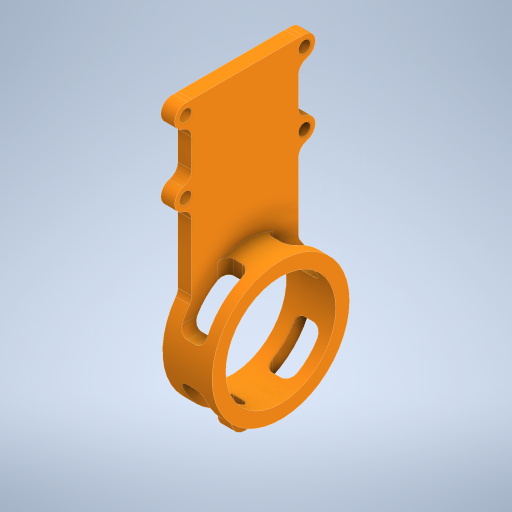
# Autodesk Inventor part: RSFF_cover_2_v2_clearance
Saved by Autodesk Inventor 2023 (Build 270158000, 158)
## iProperties
Created: 2023-10-18
Part Number: RSFF_cover_2_v2_clearance
Material: Generic
Document SubType Name: Modeling
Designer: MichihisaOohara
Density: 1 g/cm^3
Appearance: オレンジ
Author: MichihisaOohara
Autodesk Inventor part; units mm, degrees
ref_plane "YZ Plane" through (0, 0, 0) normal (1, 0, 0) x (0, 1, 0)
ref_plane "XZ Plane" through (0, 0, 0) normal (0, 1, 0) x (-1, 0, 0)
ref_plane "XY Plane" through (0, 0, 0) normal (0, 0, 1) x (1, 0, 0)
sketch "スケッチ1" plane through (0, 0, 0) normal (1, 0, 0) x (0, 1, 0)
  circle A0 centre (0, 0) radius 10
  circle A1 centre (0, 0) radius 12.5
  line L0 (24.5, 10.8) -> (37.5, 10.8)
  line L1 (37.5, 10.8) -> (37.5, -10.8)
  line L2 (37.5, -10.8) -> (24.5, -10.8)
  line L3 (24.5, -10.8) -> (24.5, 10.8)
  circle A2 centre (37.5, 10.8) radius 1.1
  circle A3 centre (37.5, -10.8) radius 1.1
  circle A4 centre (24.5, 10.8) radius 1.1
  circle A5 centre (24.5, -10.8) radius 1.1
  line L4 (0, 9.7) -> (39.5, 9.7)
  line L5 (39.5, 9.7) -> (39.5, -9.7)
  line L6 (39.5, -9.7) -> (0, -9.7)
  line L7 (0, -9.7) -> (0, 9.7)
  circle A6 centre (37.5, 10.8) radius 2
  circle A7 centre (37.5, -10.8) radius 2
  circle A8 centre (24.5, -10.8) radius 2
  circle A9 centre (24.5, 10.8) radius 2
  point P0 (7.8842, 9.7)
  point P1 (7.8842, -9.7)
  point P2 (22.8297, -9.7)
  point P3 (26.1703, -9.7)
  point P4 (35.8297, -9.7)
  point P5 (39.1703, -9.7)
  point P6 (39.1703, 9.7)
  point P7 (35.8297, 9.7)
  point P8 (26.1703, 9.7)
  point P9 (22.8297, 9.7)
  dimension "d0" = 20
  dimension "d1" = 25
  dimension "d2" = 13
  dimension "d3" = 24.5
  dimension "d4" = 10.8
  dimension "d5" = 21.6
  dimension "d6" = 2.2
  dimension "d7" = 2.2
  dimension "d8" = 2.2
  dimension "d9" = 2.2
  dimension "d10" = 19.4
  dimension "d11" = 9.7
  dimension "d12" = 2
  dimension "d13" = 0
  dimension "d14" = 4
  dimension "d15" = 4
  dimension "d16" = 4
  dimension "d17" = 4
  constraints: 16 end point, 10 centre point, 10 coincident, 4 parallel, 2 horizontal, 2 perpendicular
  measures "d0" diameter of A0
  measures "d1" diameter of A1
  measures "d2" distance of L0.start L0.end
  measures "d3" distance from line of point (0, 0) L3
  measures "d4" distance from line of point (0, 0) L0
  measures "d5" distance of L0.end L1.end
  measures "d6" diameter of A2
  measures "d7" diameter of A3
  measures "d8" diameter of A4
  measures "d9" diameter of A5
  measures "d10" distance of L4.end L5.end
  measures "d11" distance from line of A0.centre L4
  measures "d12" distance between parallel lines of L1 L5
  measures "d13" distance from line of point (0, 0) L7
  measures "d14" diameter of A6
  measures "d15" diameter of A7
  measures "d16" diameter of A9
  measures "d17" diameter of A8
extrude "押し出し1" add sketch "スケッチ1" against normal blind 2.5 contours A0 L4 A1 L6 | A0 L6 A1 L4 | L4 A9 L3 A8 L6 A1 | A9 L0 A4 L4 | L4 L3 A9 | A8 L3 L6 | L6 A5 L2 A8 | L4 A9 L3 | A4 L0 A9 L4 | A9 L4 A6 L1 A7 L6 A8 L3 | L6 A8 L2 A5 | L3 A8 L6 | A6 L4 A2 L0 | L0 A2 L4 A6 | A7 L6 A3 L2 | L2 A3 L6 A7 | L4 L1 A6 | A7 L1 L6 | L4 A6 L1 | A6 L4 L5 L6 A7 L1 | L1 A7 L6
fillet "フィレット1" radius 2 10 edges at (-1.25, 39.1703, 9.7) (-1.25, 39.1703, -9.7) (-1.25, 35.8297, 9.7) (-1.25, 35.8297, -9.7) (-1.25, 22.8297, 9.7) (-1.25, 26.1703, 9.7) (-1.25, 26.1703, -9.7) (-1.25, 22.8297, -9.7) (-1.25, 7.8842, 9.7) (-1.25, 7.8842, -9.7)
sketch "スケッチ2" plane through (0, 0, 0) normal (1, 0, 0) x (0, 0, -1)
  line L0 (-12.5, 3.5) -> (12.5, 3.5)
  line L1 (12.5, 3.5) -> (12.5, -3.5)
  line L2 (12.5, -3.5) -> (-12.5, -3.5)
  line L3 (-12.5, -3.5) -> (-12.5, 3.5)
  line L4 (-12.5, 3.5) -> (12.5, -3.5) construction
  line L5 (12.5, 3.5) -> (-12.5, -3.5) construction
  line L6 (-3.5, -12.5) -> (3.5, -12.5)
  line L7 (3.5, -12.5) -> (3.5, 12.5)
  line L8 (3.5, 12.5) -> (-3.5, 12.5)
  line L9 (-3.5, 12.5) -> (-3.5, -12.5)
  line L10 (-3.5, -12.5) -> (3.5, 12.5) construction
  line L11 (3.5, -12.5) -> (-3.5, 12.5) construction
  circle A0 centre (0, 0) radius 10
  arc A1 (-10.0862, 7.3837) -> (10.0862, 7.3837) centre (0, 0) ccw projected
  circle A2 centre (0, 0) radius 12.5
  point P0 (12, 3.5)
  point P1 (9.3675, 3.5)
  point P2 (9.3675, -3.5)
  point P3 (12, -3.5)
  point P4 (3.5, -12)
  point P5 (3.5, -9.3675)
  point P6 (-3.5, -9.3675)
  point P7 (-3.5, -12)
  point P8 (-12, 3.5)
  point P9 (-12, -3.5)
  point P10 (-9.3675, -3.5)
  point P11 (-9.3675, 3.5)
  point P12 (-3.5, 12)
  point P13 (-3.5, 9.3675)
  point P14 (3.5, 9.3675)
  point P15 (3.5, 12)
  dimension "d21" = 7
  dimension "d22" = 25
  dimension "d23" = 7
  dimension "d24" = 25
  dimension "d25" = 20
  constraints: 24 end point, 4 midpoint, 4 parallel, 2 coincident, 2 horizontal, 2 perpendicular, 1 centre point, 3 other
  measures "d21" distance of L2.end L0.start
  measures "d22" distance of L1.end L2.end
  measures "d23" distance of L7.end L8.end
  measures "d24" distance of L8.end L6.start
  measures "d25" diameter of A0
extrude "押し出し2" add sketch "スケッチ2" along normal blind 4.5 contours L0 A0 L2 A1 | L9 A2 L7 A0 | L9 A0 L7 A1 | L0 A1 L2 A0
sketch "スケッチ3" plane through (4.5, 0, 0) normal (1, 0, 0) x (0, 0, -1)
  circle A0 centre (0, 0) radius 10
  circle A1 centre (0, 0) radius 12.5
  point P0 (3.5, 12)
  dimension "d28" = 20
  constraints: 2 coincident, 1 centre point, 3 other
  measures "d28" diameter of A0
extrude "押し出し3" add sketch "スケッチ3" along normal blind 2
fillet "フィレット2" radius 1.5 8 edges at (0, 10.6837, 3.5) (0, 10.6837, -3.5) (0, 3.5, 10.6837) (0, -3.5, 10.6837) (0, -10.6837, -3.5) (0, -3.5, -10.6837) (0, 3.5, -10.6837) (0, -10.6837, 3.5)
fillet "フィレット3" radius 1.5 8 edges at (4.5, 10.6837, 3.5) (4.5, 10.6837, -3.5) (4.5, 3.5, -10.6837) (4.5, -3.5, -10.6837) (4.5, -10.6837, -3.5) (4.5, -10.6837, 3.5) (4.5, -3.5, 10.6837) (4.5, 3.5, 10.6837)
sketch "スケッチ4" plane through (-2.5, 0, 0) normal (-1, 0, 0) x (0, 0, 1)
  circle A0 centre (0, -15) radius 1.1
  circle A1 centre (0, -15) radius 2.5
  circle A2 centre (0, 0) radius 10 projected
  line L0 (2.5, -15) -> (-2.5, -15)
  line L1 (-2.5, -15) -> (-2.5, -9.6825)
  line L2 (-2.5, -9.6825) -> (2.5, -9.6825)
  line L3 (2.5, -9.6825) -> (2.5, -15)
  dimension "d35" = 5
  dimension "d33" = 15
  dimension "d34" = 2.2
  dimension "d36" = 0
  dimension "d40" = 5
  dimension "d41" = 5.3175
  constraints: 8 end point, 2 parallel, 1 centre point, 1 coincident, 1 horizontal, 1 perpendicular, 5 other
  measures "d33" distance of point (0, 0) A0.centre
  measures "d34" diameter of A0
  measures "d36" horizontal distance of point (0, 0) A0.centre
  measures "d40" distance of L0.start L0.end
  measures "d41" distance of L2.end L0.start
extrude "押し出し4" add sketch "スケッチ4" against normal blind 2.5 contours L0 A1 A0 | A0 L0 A1 | A1 L1 A2 L3
fillet "フィレット5" radius 3 2 edges at (-1.25, -12.2474, 2.5) (-1.25, -12.2474, -2.5)
equation "\"d4\" = 0.5 * d5"
equation "\"d7\" = d6"
equation "\"d8\" = d6"
equation "\"d9\" = d6"
equation "\"d11\" = 0.5 * d10"
equation "\"d15\" = d14"
equation "\"d16\" = d14"
equation "\"d17\" = d14"
equation "\"d23\" = d21"
equation "\"d24\" = d22"
equation "\"d40\" = d35"
